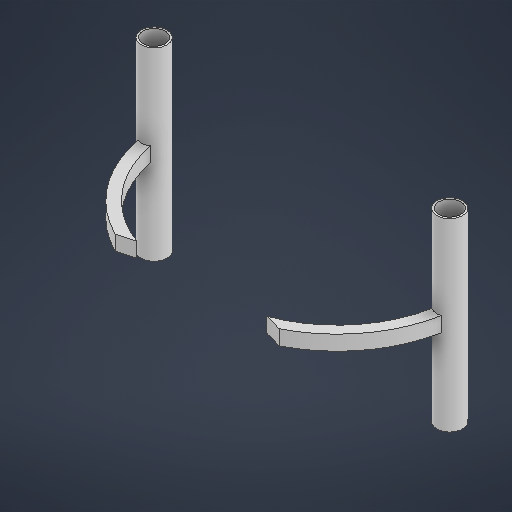
# Autodesk Inventor part: stand
Saved by Autodesk Inventor 2026.1 (Build 301233000, 233)
## iProperties
Created: 2025-09-08
Part Number: stand
Material: 일반
Document SubType Name: Modeling
Designer: ytw32
Density: 1 g/cm^3
Appearance: 기본값
Author: ytw32
Autodesk Inventor part; units mm, degrees
ref_plane "YZ Plane" through (0, 0, 0) normal (1, 0, 0) x (0, 1, 0)
ref_plane "XZ Plane" through (0, 0, 0) normal (0, 1, 0) x (-1, 0, 0)
ref_plane "XY Plane" through (0, 0, 0) normal (0, 0, 1) x (1, 0, 0)
sketch "스케치1" plane through (0, 0, 0) normal (0, 1, 0) x (-1, 0, 0)
  line L0 (0, 0) -> (-400, 0)
  circle A0 centre (-400, 0) radius 35
  circle A1 centre (-400, 0) radius 30
  line L1 (0, 0) -> (0, 250)
  arc A2 (-200, 277.1584) -> (-175.6469, 270.8579) centre (0, 1000) ccw
  line L2 (0, 0) -> (0, 300)
  arc A3 (-414.9319, 1.4273) -> (-385.0681, -1.4273) centre (-400, 0) ccw
  arc A4 (-175.6469, 270.8579) -> (-385.0681, -1.4273) centre (-63.367, -32.1773) ccw
  arc A5 (-221.6912, 283.5134) -> (-200, 277.1584) centre (0, 1000) ccw
  arc A6 (-221.6912, 283.5134) -> (-414.9319, 1.4273) centre (-63.367, -32.1773) ccw
  point P0 (-410.3883, 33.4228)
  point P1 (-380.6581, 29.17)
  dimension "d0" = 400
  dimension "d1" = 70
  dimension "d2" = 60
  dimension "d3" = 250
  dimension "d6" = 300
  constraints: 11 point on circle, 7 centre point, 6 end point, 2 coincident, 1 horizontal, 1 vertical
  measures "d0" distance of L0.start L0.end
  measures "d1" diameter of A0
  measures "d2" diameter of A1
  measures "d3" distance of L0.start L1.end
  measures "d6" distance of L0.start L2.end
extrude "돌출1" add sketch "스케치1" along normal mid plane 500 contours A0 A6 A1 L0 | L0 A1 A4 A0 | A4 A1 A6 A0
extrude "돌출2" add sketch "스케치1" along normal mid plane 40 contours A0 A6 A5 A2 A4
mirror "미러1" about plane through (0, 0, 0) normal (1, 0, 0) of "돌출1", "돌출2"
